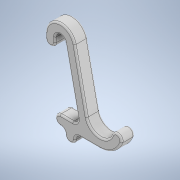
# Autodesk Inventor part: BedDowelHookV2
Saved by Autodesk Inventor 2020 (Build 240168000, 168)
## iProperties
Created: 2019-12-18
Part Number: BedDowelHookV2
Material: Generic
Document SubType Name: Modeling
Designer: Connor
Density: 1 g/cm^3
Appearance: Default
Author: Connor
Autodesk Inventor part; units mm, degrees
ref_plane "YZ Plane" through (0, 0, 0) normal (1, 0, 0) x (0, 1, 0)
ref_plane "XZ Plane" through (0, 0, 0) normal (0, 1, 0) x (-1, 0, 0)
ref_plane "XY Plane" through (0, 0, 0) normal (0, 0, 1) x (1, 0, 0)
sketch "Sketch1" plane through (0, 0, 0) normal (0, 0, 1) x (1, 0, 0)
  circle A0 centre (0, 0) radius 4.7625
  arc A1 (4.7625, -76.2) -> (0, -71.4375) centre (0, -76.2) ccw
  circle A2 centre (-9.525, -4.7625) radius 4.7625
  line L0 (-4.7625, 0) -> (-4.7625, -4.7625)
  line L1 (-14.2875, 0) -> (-14.2875, -4.7625)
  line L2 (-9.525, -4.7625) -> (0, -4.7625) construction
  circle A3 centre (0, 0) radius 14.2875 construction
  arc A4 (13.9727, 2.9825) -> (-14.2875, 0) centre (0, 0) ccw
  line L3 (13.9727, 2.9825) -> (25.6798, -51.8636)
  circle A5 centre (0, -76.2) radius 14.2875 construction
  circle A6 centre (38.1, -49.2125) radius 12.7 construction
  line L4 (38.1, -49.2125) -> (50.0341, -53.5562) construction
  line L5 (38.1, -49.2125) -> (25.4, -49.2125) construction
  circle A7 centre (54.5094, -55.185) radius 4.7625
  arc A8 (38.1, -71.4375) -> (58.9847, -56.8139) centre (38.1, -49.2125) ccw
  arc A9 (4.7625, -76.2) -> (14.2875, -76.2) centre (9.525, -76.2) ccw
  arc A10 (19.05, -71.4375) -> (14.2875, -76.2) centre (19.05, -76.2) ccw
  arc A11 (0, -61.9125) -> (0, -71.4375) centre (0, -66.675) ccw
  line L6 (-4.7625, 0) -> (-4.7625, -4.7625)
  line L7 (12.1988, -61.9125) -> (0, -61.9125)
  arc A12 (12.1988, -61.9125) -> (16.8564, -56.1558) centre (12.1988, -57.15) ccw
  line L8 (38.1, -71.4375) -> (19.05, -71.4375)
  arc A13 (25.6798, -51.8636) -> (50.0341, -53.5562) centre (38.1, -49.2125) ccw
  line L9 (25.4, 13.5278) -> (25.4, -4.2823) construction
  line L10 (4.6576, 0.9942) -> (16.8564, -56.1558)
  dimension "d0" = 9.525
  dimension "d7" = 76.2
  dimension "d10" = 160
  dimension "d12" = 38.1
  dimension "d13" = 25.4
  dimension "d17" = 25.4
  constraints: 29 point on circle, 22 end point, 20 tangent, 14 centre point, 8 equal radius, 7 coincident, 4 horizontal, 3 vertical, 1 parallel, 1 point on line, 1 vertical alignment
  measures "d0" diameter of A0
  measures "d7" distance of A1.centre point (0, 0)
  measures "d10" angle of L5 L4
  measures "d12" horizontal distance of A6.centre point (0, 0)
  measures "d13" distance from line of point (0, 0) L9
  measures "d17" diameter of A6
extrude "Extrusion1" add sketch "Sketch1" along normal blind 12.7 contours A0 L0 A2 L1 A4 L3 A13 A7 A8 L8 A10 A9 A1 A11 L7 A12 L10 | A2 | A7
fillet "Fillet1" radius 1.5875 34 edges at (15.9013, -60.1456, 12.7) (6.0994, -61.9125, 12.7) (-4.7625, -66.675, 12.7) (3.3676, -72.8324, 12.7) (9.525, -80.9625, 12.7) (15.6824, -72.8324, 12.7) (28.575, -71.4375, 12.7) (50.8477, -67.4182, 12.7) (56.1383, -50.7097, 12.7) (37.2195, -61.8819, 12.7) (19.8263, -24.4406, 12.7) (-1.4995, 14.2086, 12.7) (-14.2875, -2.3813, 12.7) (-9.525, -9.525, 12.7) (-4.7625, -2.3813, 12.7) (-0.4998, 4.7362, 12.7) (10.757, -27.5808, 12.7) (15.9013, -60.1456, 0) (6.0994, -61.9125, 0) (-4.7625, -66.675, 0) (3.3676, -72.8324, 0) (9.525, -80.9625, 0) (15.6824, -72.8324, 0) (28.575, -71.4375, 0) (50.8477, -67.4182, 0) (56.1383, -50.7097, 0) (37.2195, -61.8819, 0) (19.8263, -24.4406, 0) (-1.4995, 14.2086, 0) (-14.2875, -2.3813, 0) (-9.525, -9.525, 0) (-4.7625, -2.3813, 0) (-0.4998, 4.7362, 0) (10.757, -27.5808, 0)
body "Solid1"
